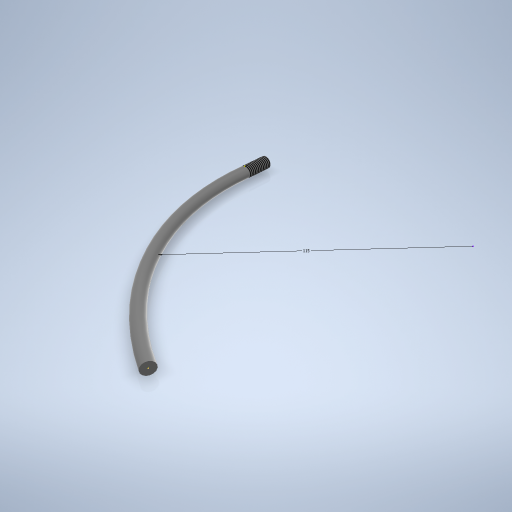
# Autodesk Inventor part: stand
Saved by Autodesk Inventor 2024.2 (Build 282272000, 272)
## iProperties
Created: 2024-05-15
Part Number: stand
Material: Acetalharz, Schwarz
Document SubType Name: Modeling
Designer: Fabri
Density: 1.425 g/cm^3
Appearance: Glatt - Schwarz
Author: Fabri
Autodesk Inventor part; units mm, degrees
ref_plane "YZ Plane" through (0, 0, 0) normal (1, 0, 0) x (0, 1, 0)
ref_plane "XZ Plane" through (0, 0, 0) normal (0, 1, 0) x (-1, 0, 0)
ref_plane "XY Plane" through (0, 0, 0) normal (0, 0, 1) x (1, 0, 0)
sketch "Skizze2" plane through (0, 0, 0) normal (0, 1, 0) x (-1, 0, 0)
  circle A0 centre (0, 0) radius 3
  dimension "d1" = 6
  constraints: 1 centre point, 1 coincident
  measures "d1" diameter of A0
sketch "Skizze3" plane through (0, 0, 0) normal (0, 0, 1) x (1, 0, 0)
  arc A0 (0, -13) -> (67, -120) centre (114.9732, -15.4841) ccw
  line L0 (0, 0) -> (0, -13)
  dimension "d2" = 115
  dimension "d3" = 120
  dimension "d4" = 67
  dimension "d8" = 13
  constraints: 2 end point, 2 point on circle, 1 centre point, 1 vertical
  measures "d2" radius of A0
  measures "d3" vertical distance of A0.end L0.start
  measures "d4" horizontal distance of A0.end L0.start
  measures "d8" distance of L0.start L0.end
sweep "Sweeping1" add profiles "Skizze2" path "Skizze3"
thread "Gewinde1"
sketch3d "3D-Skizze2"
